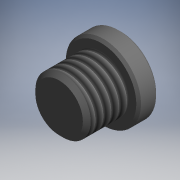
# Autodesk Inventor part: Verschlussschraube DIN908 M7
Saved by Autodesk Inventor 2017.3 (Build 213256000, 256)
## iProperties
Part Number: Verschlussschraube DIN908 M7
Material: Generic
Catalog Web Link: www.cadenas.de
Description: DIN 908-Verschlußschraube
Vendor: SCHUNK
Document SubType Name: Modeling
Designer: partserver
Manufacturer: SCHUNK
Mass: 0.35644 g
Surface Area: 3.41421 cm^2
Volume: 0.35644 cm^3
Density: 1 g/cm^3
Appearance: PSOLRGB-128-128-128
Category: PARTsolutions
Company: SCHUNK
Title: Verschlussschraube DIN908 M7
Author: Cadenas PARTsolutions
Comments: Verschlußschraube
PSOL_IDENT_0: {$CADENAS_DATA\23d-libs\schunk\normteile\din_908_verschlussschraube.prj},198 {VTYP=3D},{NB=Verschlus
PSOL_IDENT_1: sschraube DIN908 M7},{LINA=Verschlussschraube DIN908 M7},{NN=DIN 908},{DATE=20.01.2020 07:52:32},{GE
PSOL_IDENT_2: OMDATE=04.12.2019 08:07:47},{VERSION=},{LINEID=370},{WBVAR=},{WBNUMERIC=}  {NB=Verschlussschraube DI
PSOL_IDENT_3: N908 M7},{LINA=Verschlussschraube DIN908 M7},{KT=DUMMY},{TYP=DIN908 M7},{TYP1=20.000},{M1=7.000},{GL=
PSOL_IDENT_4: 5.300},{SK=9.500},{SKH=2.500},{SW=3.000},{SWT=2.500}
NB: Verschlussschraube DIN908 M7
NN: DIN 908
NT: Verschlußschraube
NBSYN: Verschlussschraube $TYP.
LINA: Verschlussschraube DIN908 M7
CATALOG: SCHUNK
TYP: DIN908 M7
TYP1: 20
SUPPLIER: SCHUNK
ARTICLENO: Verschlussschraube DIN908 M7
BOMINFO: Verschlussschraube DIN908 M7
CREATOR: CADENAS GmbH
Autodesk Inventor part; units mm, degrees
sketch "Sketch_1" plane through (0, 0, 0) normal (0, 0, 1) x (1, 0, 0)
  line L0 (0, -5.3) -> (0, 2.5)
  line L1 (0, 2.5) -> (4.45, 2.5)
  line L2 (4.45, 2.5) -> (4.75, 2.2)
  line L3 (4.75, 2.2) -> (4.75, 0.3)
  line L4 (4.75, 0.3) -> (4.45, 0)
  line L5 (4.45, 0) -> (3.5, 0)
  line L6 (3.5, 0) -> (3.5, -4.8)
  line L7 (3.5, -4.8) -> (3, -5.3)
  line L8 (3, -5.3) -> (0, -5.3)
  line L9 (0, -5.3) -> (0, 2.5)
  constraints: 20 end point
revolve "Revolution1" add sketch "Sketch_1" angle 360 about axis through (0, -5.3, 0) along (0, -1, 0)
thread "Thread1" size "M7x1" class "6g" standard "ISO Metric profile" full length
sketch "Sketch_4" plane through (0, 2.5, 0) normal (0, 1, 0) x (1, 0, 0)
  line L0 (-1.5, -0.866) -> (0, -1.7321)
  line L1 (0, -1.7321) -> (1.5, -0.866)
  line L2 (1.5, -0.866) -> (1.5, 0.866)
  line L3 (1.5, 0.866) -> (0, 1.7321)
  line L4 (0, 1.7321) -> (-1.5, 0.866)
  line L5 (-1.5, 0.866) -> (-1.5, -0.866)
  constraints: 12 end point
extrude "Extrusion1" cut sketch "Sketch_4" against normal blind 2.5
ref_plane "din_908_XY" through (0, 0, 0) normal (0, 1, 0) x (1, 0, 0)
ref_plane "din_908_YZ" through (0, 0, 0) normal (1, 0, 0) x (0, 0, -1)
ref_plane "din_908_ZX" through (0, 0, 0) normal (0, 0, -1) x (0, 1, 0)
body "Solid1"
